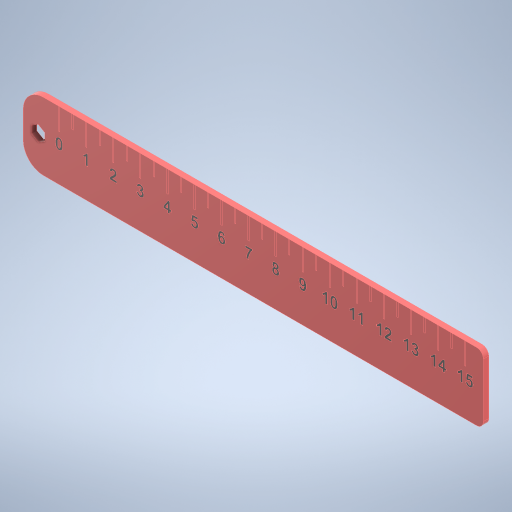
# Autodesk Inventor part: Regua
Saved by Autodesk Inventor 2023 (Build 270158000, 158)
## iProperties
Created: 2024-09-26
Part Number: Regua
Material: Acrílico
Document SubType Name: Modeling
Designer: Aluno
Density: 1.188 g/cm^3
Appearance: Suave - Vermelho
Author: Aluno
Autodesk Inventor part; units mm, degrees
ref_plane "YZ Plane" through (0, 0, 0) normal (1, 0, 0) x (0, 1, 0)
ref_plane "XZ Plane" through (0, 0, 0) normal (0, 1, 0) x (-1, 0, 0)
ref_plane "XY Plane" through (0, 0, 0) normal (0, 0, 1) x (1, 0, 0)
sketch "Esboço1" plane through (0, 0, 0) normal (0, 0, 1) x (1, 0, 0)
  line L0 (-85, 12.5) -> (85, 12.5)
  line L1 (85, 12.5) -> (85, -12.5)
  line L2 (85, -12.5) -> (-85, -12.5)
  line L3 (-85, -12.5) -> (-85, 12.5)
  point P0 (0, 0)
  point P1 (-85, 0)
  point P2 (0, 12.5)
  dimension "d0" = 170
  dimension "d1" = 25
  constraints: 8 end point, 2 midpoint, 2 parallel, 1 horizontal, 1 horizontal alignment, 1 perpendicular, 1 vertical alignment
  measures "d0" distance of L0.start L0.end
  measures "d1" distance of L0.end L1.end
extrude "Extrusão1" add sketch "Esboço1" along normal mid plane 2
fillet "Arredondamento3" radius 7.5 2 edges at (-85, -12.5, 0) (-85, 12.5, 0)
sketch "Esboço3" plane through (0, 0, 1) normal (0, 0, 1) x (1, 0, 0)
  line L0 (-72, 12.5) -> (-71.5, 12.5)
  line L1 (-71.5, 12.5) -> (-71.5, 4.5)
  line L2 (-71.5, 4.5) -> (-72, 4.5)
  line L3 (-72, 4.5) -> (-72, 12.5)
  line L4 (85, 12.5) -> (-77.5, 12.5) projected
  line L5 (-85, 5) -> (-85, -5) projected
  line L6 (-77.5, 12.5) -> (85, 12.5) projected
  line L7 (-67, 12.5) -> (-66.5, 12.5)
  line L8 (-66.5, 12.5) -> (-66.5, 7.5)
  line L9 (-66.5, 7.5) -> (-67, 7.5)
  line L10 (-67, 7.5) -> (-67, 12.5)
  point P0 (0, 0)
  point P1 (72.75, 12.5)
  point P2 (-71.75, 12.5)
  point P3 (-2.375, 12.5)
  point P4 (-66.75, 12.5)
  dimension "d11" = 0.5
  dimension "d12" = 8
  dimension "d13" = 13
  dimension "d14" = 5
  dimension "d15" = 5
  constraints: 16 end point, 5 parallel, 2 horizontal, 2 midpoint, 2 perpendicular, 2 point on line, 1 horizontal alignment
  measures "d11" distance between parallel lines of L3 L1
  measures "d12" distance of L2.end L0.start
  measures "d13" distance between parallel lines of L5 L3
  measures "d14" distance of L9.end L7.start
  measures "d15" distance of point (-71.75, 12.5) point (-66.75, 12.5)
extrude "Extrusão3" cut sketch "Esboço3" against normal blind 0.001
pattern_linear "Padrão retangular1" count 16 spacing 10 along (1, 0, 0) of "Extrusão3"
sketch "Esboço5" plane through (0, 0, 1) normal (0, 0, 1) x (1, 0, 0)
  line L0 (-77, -1.4434) -> (-79.5, -2.8868)
  line L1 (-79.5, -2.8868) -> (-82, -1.4434)
  line L2 (-82, -1.4434) -> (-82, 1.4434)
  line L3 (-82, 1.4434) -> (-79.5, 2.8868)
  line L4 (-79.5, 2.8868) -> (-77, 1.4434)
  line L5 (-77, 1.4434) -> (-77, -1.4434)
  line L6 (-85, 5) -> (-85, -5) projected
  point P0 (0, 0)
  point P1 (-79.5, 0)
  dimension "d23" = 5
  dimension "d24" = 5.5
  constraints: 12 end point, 1 horizontal alignment, 1 vertical alignment, 13 other
  measures "d23" distance between parallel lines of L2 L5
  measures "d24" distance from line of L6 point (-79.5, 0)
extrude "Extrusão5" cut sketch "Esboço5" against normal up to surface (2 mm away)
sketch "Esboço7" plane through (0, 0, 1) normal (0, 0, 1) x (1, 0, 0)
  line L0 (-74.25, 2.5) -> (-69.25, 2.5) construction
  line L1 (-69.25, 2.5) -> (-69.25, -1.5) construction
  line L2 (-69.25, -1.5) -> (-74.25, -1.5) construction
  line L3 (-74.25, -1.5) -> (-74.25, 2.5) construction
  line L4 (-71.5, 4.5) -> (-72, 4.5) projected
  line L5 (-64.25, 2.5) -> (-59.25, 2.5) construction
  line L6 (-59.25, 2.5) -> (-59.25, -1.5) construction
  line L7 (-59.25, -1.5) -> (-64.25, -1.5) construction
  line L8 (-64.25, -1.5) -> (-64.25, 2.5) construction
  line L9 (-54.25, 2.5) -> (-49.25, 2.5) construction
  line L10 (-49.25, 2.5) -> (-49.25, -1.5) construction
  line L11 (-49.25, -1.5) -> (-54.25, -1.5) construction
  line L12 (-54.25, -1.5) -> (-54.25, 2.5) construction
  line L13 (-44.25, 2.5) -> (-39.25, 2.5) construction
  line L14 (-39.25, 2.5) -> (-39.25, -1.5) construction
  line L15 (-39.25, -1.5) -> (-44.25, -1.5) construction
  line L16 (-44.25, -1.5) -> (-44.25, 2.5) construction
  line L17 (-34.25, -1.5) -> (-34.25, 2.5) construction
  line L18 (-34.25, 2.5) -> (-29.25, 2.5) construction
  line L19 (-29.25, 2.5) -> (-29.25, -1.5) construction
  line L20 (-29.25, -1.5) -> (-34.25, -1.5) construction
  line L21 (-24.25, -1.5) -> (-24.25, 2.5) construction
  line L22 (-24.25, 2.5) -> (-19.25, 2.5) construction
  line L23 (-19.25, 2.5) -> (-19.25, -1.5) construction
  line L24 (-19.25, -1.5) -> (-24.25, -1.5) construction
  line L25 (-14.25, -1.5) -> (-14.25, 2.5) construction
  line L26 (-14.25, 2.5) -> (-9.25, 2.5) construction
  line L27 (-9.25, 2.5) -> (-9.25, -1.5) construction
  line L28 (-9.25, -1.5) -> (-14.25, -1.5) construction
  line L29 (-4.25, -1.5) -> (-4.25, 2.5) construction
  line L30 (-4.25, 2.5) -> (0.75, 2.5) construction
  line L31 (0.75, 2.5) -> (0.75, -1.5) construction
  line L32 (0.75, -1.5) -> (-4.25, -1.5) construction
  line L33 (5.75, -1.5) -> (5.75, 2.5) construction
  line L34 (5.75, 2.5) -> (10.75, 2.5) construction
  line L35 (10.75, 2.5) -> (10.75, -1.5) construction
  line L36 (10.75, -1.5) -> (5.75, -1.5) construction
  line L37 (15.75, -1.5) -> (15.75, 2.5) construction
  line L38 (15.75, 2.5) -> (20.75, 2.5) construction
  line L39 (20.75, 2.5) -> (20.75, -1.5) construction
  line L40 (20.75, -1.5) -> (15.75, -1.5) construction
  line L41 (25.75, -1.5) -> (25.75, 2.5) construction
  line L42 (25.75, 2.5) -> (30.75, 2.5) construction
  line L43 (30.75, 2.5) -> (30.75, -1.5) construction
  line L44 (30.75, -1.5) -> (25.75, -1.5) construction
  line L45 (35.75, -1.5) -> (35.75, 2.5) construction
  line L46 (35.75, 2.5) -> (40.75, 2.5) construction
  line L47 (40.75, 2.5) -> (40.75, -1.5) construction
  line L48 (40.75, -1.5) -> (35.75, -1.5) construction
  line L49 (45.75, -1.5) -> (45.75, 2.5) construction
  line L50 (45.75, 2.5) -> (50.75, 2.5) construction
  line L51 (50.75, 2.5) -> (50.75, -1.5) construction
  line L52 (50.75, -1.5) -> (45.75, -1.5) construction
  line L53 (55.75, -1.5) -> (55.75, 2.5) construction
  line L54 (55.75, 2.5) -> (60.75, 2.5) construction
  line L55 (60.75, 2.5) -> (60.75, -1.5) construction
  line L56 (60.75, -1.5) -> (55.75, -1.5) construction
  line L57 (65.75, -1.5) -> (65.75, 2.5) construction
  line L58 (65.75, 2.5) -> (70.75, 2.5) construction
  line L59 (70.75, 2.5) -> (70.75, -1.5) construction
  line L60 (70.75, -1.5) -> (65.75, -1.5) construction
  line L61 (68.5, 4.5) -> (68, 4.5) projected
  line L62 (58.5, 4.5) -> (58, 4.5) projected
  line L63 (48.5, 4.5) -> (48, 4.5) projected
  line L64 (38.5, 4.5) -> (38, 4.5) projected
  line L65 (28.5, 4.5) -> (28, 4.5) projected
  line L66 (18.5, 4.5) -> (18, 4.5) projected
  line L67 (8.5, 4.5) -> (8, 4.5) projected
  line L68 (-1.5, 4.5) -> (-2, 4.5) projected
  line L69 (-11.5, 4.5) -> (-12, 4.5) projected
  line L70 (-21.5, 4.5) -> (-22, 4.5) projected
  line L71 (75.75, -1.5) -> (75.75, 2.5) construction
  line L72 (75.75, 2.5) -> (80.75, 2.5) construction
  line L73 (80.75, 2.5) -> (80.75, -1.5) construction
  line L74 (80.75, -1.5) -> (75.75, -1.5) construction
  line L75 (78.5, 4.5) -> (78, 4.5) projected
  line L76 (-61.5, 4.5) -> (-62, 4.5) projected
  line L77 (-51.5, 4.5) -> (-52, 4.5) projected
  line L78 (-41.5, 4.5) -> (-42, 4.5) projected
  line L79 (-31.5, 4.5) -> (-32, 4.5) projected
  spline S0 degree 2 poles (-71.7698, 2.5412) (-71.1875, 2.5412) (-70.8613, 2.1265) knots 0 0 0 1 1 1
  spline S1 degree 2 poles (-70.8613, 2.1265) (-70.471, 1.6357) (-70.471, 0.4985) knots 0 0 0 1 1 1
  spline S2 degree 2 poles (-70.471, 0.4985) (-70.471, -0.6357) (-70.8643, -1.1326) knots 0 0 0 1 1 1
  spline S3 degree 2 poles (-70.8643, -1.1326) (-71.1875, -1.5412) (-71.7698, -1.5412) knots 0 0 0 1 1 1
  spline S4 degree 2 poles (-71.7698, -1.5412) (-72.3552, -1.5412) (-73.0686, -0.6448) (-73.0686, 0.5076) knots 0 0 0 1 2 2 2
  spline S5 degree 2 poles (-73.0686, 0.5076) (-73.0686, 1.6357) (-72.6753, 2.1326) knots 0 0 0 1 1 1
  spline S6 degree 2 poles (-72.6753, 2.1326) (-72.3521, 2.5412) (-71.7698, 2.5412) knots 0 0 0 1 1 1
  spline S7 degree 2 poles (-71.7698, 1.904) (-71.9101, 1.904) (-72.1265, 1.7271) (-72.1875, 1.4985) knots 0 0 0 1 2 2 2
  spline S8 degree 2 poles (-72.1875, 1.4985) (-72.2668, 1.2027) (-72.2668, 0.4985) knots 0 0 0 1 1 1
  spline S9 degree 2 poles (-72.2668, 0.4985) (-72.2668, -0.2027) (-72.1235, -0.7302) (-71.9101, -0.904) (-71.7698, -0.904) knots 0 0 0 1 2 3 3 3
  spline S10 degree 2 poles (-71.7698, -0.904) (-71.6296, -0.904) (-71.4131, -0.7271) (-71.3521, -0.4985) knots 0 0 0 1 2 2 2
  spline S11 degree 2 poles (-71.3521, -0.4985) (-71.2729, -0.2027) (-71.2729, 0.4985) knots 0 0 0 1 1 1
  spline S12 degree 2 poles (-71.2729, 0.4985) (-71.2729, 1.2027) (-71.4162, 1.7271) (-71.6296, 1.904) (-71.7698, 1.904) knots 0 0 0 1 2 3 3 3
  line L80 (-61.1021, -1.5076) -> (-61.8704, -1.5076)
  line L81 (-61.8704, -1.5076) -> (-61.8704, 1.3796)
  spline S13 degree 2 poles (-61.8704, 1.3796) (-62.2912, 0.9893) (-62.8613, 0.8003) knots 0 0 0 1 1 1
  line L82 (-62.8613, 0.8003) -> (-62.8613, 1.4954)
  spline S14 degree 2 poles (-62.8613, 1.4954) (-62.5595, 1.593) (-61.8552, 2.1418) (-61.7241, 2.5076) knots 0 0 0 1 2 2 2
  line L83 (-61.7241, 2.5076) -> (-61.1021, 2.5076)
  line L84 (-61.1021, 2.5076) -> (-61.1021, -1.5076)
  line L85 (-50.4771, -0.7942) -> (-50.4771, -1.5076)
  line L86 (-50.4771, -1.5076) -> (-53.1631, -1.5076)
  spline S15 degree 2 poles (-53.1631, -1.5076) (-53.1204, -1.1052) (-52.6845, -0.3826) (-52.0381, 0.2149) knots 0 0 0 1 2 2 2
  spline S16 degree 2 poles (-52.0381, 0.2149) (-51.5198, 0.6966) (-51.404, 0.8704) knots 0 0 0 1 1 1
  spline S17 degree 2 poles (-51.404, 0.8704) (-51.2454, 1.1082) (-51.2454, 1.3399) knots 0 0 0 1 1 1
  spline S18 degree 2 poles (-51.2454, 1.3399) (-51.2454, 1.596) (-51.5198, 1.8704) (-51.7637, 1.8704) knots 0 0 0 1 2 2 2
  spline S19 degree 2 poles (-51.7637, 1.8704) (-52.0015, 1.8704) (-52.2851, 1.5808) (-52.3064, 1.2454) knots 0 0 0 1 2 2 2
  line L87 (-52.3064, 1.2454) -> (-53.0716, 1.3216)
  spline S20 degree 2 poles (-53.0716, 1.3216) (-53.0046, 1.9558) (-52.2851, 2.5076) (-51.7454, 2.5076) knots 0 0 0 1 2 2 2
  spline S21 degree 2 poles (-51.7454, 2.5076) (-51.154, 2.5076) (-50.4771, 1.8704) (-50.4771, 1.3948) knots 0 0 0 1 2 2 2
  spline S22 degree 2 poles (-50.4771, 1.3948) (-50.4771, 1.1265) (-50.6692, 0.6387) (-50.8796, 0.3704) knots 0 0 0 1 2 2 2
  spline S23 degree 2 poles (-50.8796, 0.3704) (-51.0198, 0.1936) (-51.7454, -0.471) (-51.9405, -0.6905) (-51.9985, -0.7942) knots 0 0 0 1 2 3 3 3
  line L88 (-51.9985, -0.7942) -> (-50.4771, -0.7942)
  line L89 (-43.093, -0.4101) -> (-42.3521, -0.3186)
  spline S24 degree 2 poles (-42.3521, -0.3186) (-42.3155, -0.6021) (-42.0046, -0.904) (-41.7851, -0.904) knots 0 0 0 1 2 2 2
  spline S25 degree 2 poles (-41.7851, -0.904) (-41.5473, -0.904) (-41.2241, -0.5442) (-41.2241, -0.2393) knots 0 0 0 1 2 2 2
  spline S26 degree 2 poles (-41.2241, -0.2393) (-41.2241, 0.0503) (-41.532, 0.3887) (-41.7546, 0.3887) knots 0 0 0 1 2 2 2
  spline S27 degree 2 poles (-41.7546, 0.3887) (-41.9009, 0.3887) (-42.1052, 0.3308) knots 0 0 0 1 1 1
  line L90 (-42.1052, 0.3308) -> (-42.0198, 0.9558)
  spline S28 degree 2 poles (-42.0198, 0.9558) (-41.7088, 0.9466) (-41.3826, 1.2332) (-41.3826, 1.471) knots 0 0 0 1 2 2 2
  spline S29 degree 2 poles (-41.3826, 1.471) (-41.3826, 1.6723) (-41.6235, 1.9101) (-41.8216, 1.9101) knots 0 0 0 1 2 2 2
  spline S30 degree 2 poles (-41.8216, 1.9101) (-42.0198, 1.9101) (-42.2973, 1.6387) (-42.3277, 1.3765) knots 0 0 0 1 2 2 2
  line L91 (-42.3277, 1.3765) -> (-43.0351, 1.4954)
  spline S31 degree 2 poles (-43.0351, 1.4954) (-42.9619, 1.8582) (-42.6631, 2.2942) (-42.1326, 2.5412) (-41.8003, 2.5412) knots 0 0 0 1 2 3 3 3
  spline S32 degree 2 poles (-41.8003, 2.5412) (-41.2363, 2.5412) (-40.8948, 2.1814) knots 0 0 0 1 1 1
  spline S33 degree 2 poles (-40.8948, 2.1814) (-40.6143, 1.8887) (-40.6143, 1.5168) knots 0 0 0 1 1 1
  spline S34 degree 2 poles (-40.6143, 1.5168) (-40.6143, 0.9924) (-41.1905, 0.6784) knots 0 0 0 1 1 1
  spline S35 degree 2 poles (-41.1905, 0.6784) (-40.846, 0.6052) (-40.4375, 0.0899) (-40.4375, -0.2729) knots 0 0 0 1 2 2 2
  spline S36 degree 2 poles (-40.4375, -0.2729) (-40.4375, -0.8003) (-41.2058, -1.5412) (-41.779, -1.5412) knots 0 0 0 1 2 2 2
  spline S37 degree 2 poles (-41.779, -1.5412) (-42.3216, -1.5412) (-43.0351, -0.9162) (-43.093, -0.4101) knots 0 0 0 1 2 2 2
  line L92 (-31.5625, -1.5076) -> (-31.5625, -0.7027)
  line L93 (-31.5625, -0.7027) -> (-33.1997, -0.7027)
  line L94 (-33.1997, -0.7027) -> (-33.1997, -0.0351)
  line L95 (-33.1997, -0.0351) -> (-31.4649, 2.5076)
  line L96 (-31.4649, 2.5076) -> (-30.8216, 2.5076)
  line L97 (-30.8216, 2.5076) -> (-30.8216, -0.032)
  line L98 (-30.8216, -0.032) -> (-30.3247, -0.032)
  line L99 (-30.3247, -0.032) -> (-30.3247, -0.7027)
  line L100 (-30.3247, -0.7027) -> (-30.8216, -0.7027)
  line L101 (-30.8216, -0.7027) -> (-30.8216, -1.5076)
  line L102 (-30.8216, -1.5076) -> (-31.5625, -1.5076)
  line L103 (-31.5625, -0.032) -> (-31.5625, 1.3369)
  line L104 (-31.5625, 1.3369) -> (-32.4832, -0.032)
  line L105 (-32.4832, -0.032) -> (-31.5625, -0.032)
  line L106 (-23.0564, -0.4131) -> (-22.2912, -0.3338)
  spline S38 degree 2 poles (-22.2912, -0.3338) (-22.2576, -0.593) (-21.9375, -0.8948) (-21.7271, -0.8948) knots 0 0 0 1 2 2 2
  spline S39 degree 2 poles (-21.7271, -0.8948) (-21.4863, -0.8948) (-21.154, -0.5046) (-21.154, -0.1082) knots 0 0 0 1 2 2 2
  spline S40 degree 2 poles (-21.154, -0.1082) (-21.154, 0.2607) (-21.4863, 0.6296) (-21.7515, 0.6296) knots 0 0 0 1 2 2 2
  spline S41 degree 2 poles (-21.7515, 0.6296) (-22.0808, 0.6296) (-22.343, 0.3369) knots 0 0 0 1 1 1
  line L107 (-22.343, 0.3369) -> (-22.9649, 0.4284)
  line L108 (-22.9649, 0.4284) -> (-22.5716, 2.5076)
  line L109 (-22.5716, 2.5076) -> (-20.5412, 2.5076)
  line L110 (-20.5412, 2.5076) -> (-20.5412, 1.7912)
  line L111 (-20.5412, 1.7912) -> (-21.9893, 1.7912)
  line L112 (-21.9893, 1.7912) -> (-22.1113, 1.1113)
  spline S42 degree 2 poles (-22.1113, 1.1113) (-21.8552, 1.2393) (-21.5869, 1.2393) knots 0 0 0 1 1 1
  spline S43 degree 2 poles (-21.5869, 1.2393) (-21.0747, 1.2393) (-20.3643, 0.4954) (-20.3643, -0.096) knots 0 0 0 1 2 2 2
  spline S44 degree 2 poles (-20.3643, -0.096) (-20.3643, -0.5899) (-20.6509, -0.9771) knots 0 0 0 1 1 1
  spline S45 degree 2 poles (-20.6509, -0.9771) (-21.0412, -1.5076) (-21.7363, -1.5076) knots 0 0 0 1 1 1
  spline S46 degree 2 poles (-21.7363, -1.5076) (-22.2881, -1.5076) (-22.9893, -0.9131) (-23.0564, -0.4131) knots 0 0 0 1 2 2 2
  line L113 (-10.468, 1.5473) -> (-11.2088, 1.4649)
  spline S47 degree 2 poles (-11.2088, 1.4649) (-11.2363, 1.6936) (-11.4649, 1.9101) (-11.6479, 1.9101) knots 0 0 0 1 2 2 2
  spline S48 degree 2 poles (-11.6479, 1.9101) (-11.8918, 1.9101) (-12.2271, 1.4741) (-12.2698, 0.7851) knots 0 0 0 1 2 2 2
  spline S49 degree 2 poles (-12.2698, 0.7851) (-11.9863, 1.1235) (-11.5595, 1.1235) knots 0 0 0 1 1 1
  spline S50 degree 2 poles (-11.5595, 1.1235) (-11.0808, 1.1235) (-10.3948, 0.3918) (-10.3948, -0.1845) knots 0 0 0 1 2 2 2
  spline S51 degree 2 poles (-10.3948, -0.1845) (-10.3948, -0.8003) (-11.1143, -1.5412) (-11.6784, -1.5412) knots 0 0 0 1 2 2 2
  spline S52 degree 2 poles (-11.6784, -1.5412) (-12.2851, -1.5412) (-13.0655, -0.5991) (-13.0655, 0.471) knots 0 0 0 1 2 2 2
  spline S53 degree 2 poles (-13.0655, 0.471) (-13.0655, 1.5716) (-12.2515, 2.5412) (-11.6021, 2.5412) knots 0 0 0 1 2 2 2
  spline S54 degree 2 poles (-11.6021, 2.5412) (-11.1479, 2.5412) (-10.5503, 2.032) (-10.468, 1.5473) knots 0 0 0 1 2 2 2
  spline S55 degree 2 poles (-12.2058, -0.1235) (-12.2058, -0.4985) (-11.8613, -0.904) (-11.6418, -0.904) knots 0 0 0 1 2 2 2
  spline S56 degree 2 poles (-11.6418, -0.904) (-11.4284, -0.904) (-11.1448, -0.5716) (-11.1448, -0.1936) knots 0 0 0 1 2 2 2
  spline S57 degree 2 poles (-11.1448, -0.1936) (-11.1448, 0.1966) (-11.4497, 0.5595) (-11.6784, 0.5595) knots 0 0 0 1 2 2 2
  spline S58 degree 2 poles (-11.6784, 0.5595) (-11.9009, 0.5595) (-12.2058, 0.2119) (-12.2058, -0.1235) knots 0 0 0 1 2 2 2
  line L114 (-3.0655, 1.7607) -> (-3.0655, 2.4741)
  line L115 (-3.0655, 2.4741) -> (-0.4436, 2.4741)
  line L116 (-0.4436, 2.4741) -> (-0.4436, 1.9162)
  spline S59 degree 2 poles (-0.4436, 1.9162) (-0.7668, 1.596) (-1.4375, 0.4009) (-1.7912, -0.9436) (-1.7881, -1.4741) knots 0 0 0 1 2 3 3 3
  line L117 (-1.7881, -1.4741) -> (-2.529, -1.4741)
  spline S60 degree 2 poles (-2.529, -1.4741) (-2.5107, -0.6448) (-1.8613, 1.0808) (-1.3216, 1.7607) knots 0 0 0 1 2 2 2
  line L118 (-1.3216, 1.7607) -> (-3.0655, 1.7607)
  spline S61 degree 2 poles (7.5899, 0.686) (7.2942, 0.811) (7.0229, 1.25) (7.0229, 1.5122) knots 0 0 0 1 2 2 2
  spline S62 degree 2 poles (7.0229, 1.5122) (7.0229, 1.9604) (7.6479, 2.5427) (8.2241, 2.5427) knots 0 0 0 1 2 2 2
  spline S63 degree 2 poles (8.2241, 2.5427) (8.7942, 2.5427) (9.4253, 1.9604) (9.4253, 1.5122) knots 0 0 0 1 2 2 2
  spline S64 degree 2 poles (9.4253, 1.5122) (9.4253, 1.2348) (9.1357, 0.8018) (8.8735, 0.686) knots 0 0 0 1 2 2 2
  spline S65 degree 2 poles (8.8735, 0.686) (9.2058, 0.5518) (9.5534, 0.0396) (9.5534, -0.2957) knots 0 0 0 1 2 2 2
  spline S66 degree 2 poles (9.5534, -0.2957) (9.5534, -0.8506) (8.846, -1.5427) (8.2607, -1.5427) knots 0 0 0 1 2 2 2
  spline S67 degree 2 poles (8.2607, -1.5427) (7.7149, -1.5427) (7.3521, -1.2561) knots 0 0 0 1 1 1
  spline S68 degree 2 poles (7.3521, -1.2561) (6.9223, -0.9177) (6.9223, -0.3293) knots 0 0 0 1 1 1
  spline S69 degree 2 poles (6.9223, -0.3293) (6.9223, -0.003) (7.2454, 0.5396) (7.5899, 0.686) knots 0 0 0 1 2 2 2
  spline S70 degree 2 poles (7.6784, -0.2561) (7.6784, -0.5732) (8.0015, -0.9268) (8.2454, -0.9268) knots 0 0 0 1 2 2 2
  spline S71 degree 2 poles (8.2454, -0.9268) (8.4832, -0.9268) (8.7942, -0.5854) (8.7942, -0.2622) knots 0 0 0 1 2 2 2
  spline S72 degree 2 poles (8.7942, -0.2622) (8.7942, 0.0183) (8.4771, 0.3598) (8.2363, 0.3598) knots 0 0 0 1 2 2 2
  spline S73 degree 2 poles (8.2363, 0.3598) (7.9527, 0.3598) (7.6784, -0.0274) (7.6784, -0.2561) knots 0 0 0 1 2 2 2
  spline S74 degree 2 poles (7.7485, 1.4573) (7.7485, 1.2287) (8.0076, 0.9726) (8.2241, 0.9726) knots 0 0 0 1 2 2 2
  spline S75 degree 2 poles (8.2241, 0.9726) (8.4436, 0.9726) (8.7058, 1.2317) (8.7058, 1.4604) knots 0 0 0 1 2 2 2
  spline S76 degree 2 poles (8.7058, 1.4604) (8.7058, 1.6738) (8.4466, 1.9329) (8.2332, 1.9329) knots 0 0 0 1 2 2 2
  spline S77 degree 2 poles (8.2332, 1.9329) (8.0107, 1.9329) (7.7485, 1.6707) (7.7485, 1.4573) knots 0 0 0 1 2 2 2
  line L119 (16.9497, -0.5427) -> (17.6905, -0.4604)
  spline S78 degree 2 poles (17.6905, -0.4604) (17.718, -0.686) (17.9466, -0.9055) (18.1357, -0.9055) knots 0 0 0 1 2 2 2
  spline S79 degree 2 poles (18.1357, -0.9055) (18.3735, -0.9055) (18.7058, -0.4695) (18.7515, 0.2195) knots 0 0 0 1 2 2 2
  spline S80 degree 2 poles (18.7515, 0.2195) (18.4649, -0.1159) (18.029, -0.1159) knots 0 0 0 1 1 1
  spline S81 degree 2 poles (18.029, -0.1159) (17.5595, -0.1159) (16.8735, 0.6098) (16.8735, 1.1921) knots 0 0 0 1 2 2 2
  spline S82 degree 2 poles (16.8735, 1.1921) (16.8735, 1.7988) (17.596, 2.5427) (18.157, 2.5427) knots 0 0 0 1 2 2 2
  spline S83 degree 2 poles (18.157, 2.5427) (18.7637, 2.5427) (19.5442, 1.6006) (19.5442, 0.5244) knots 0 0 0 1 2 2 2
  spline S84 degree 2 poles (19.5442, 0.5244) (19.5442, -0.5732) (18.7302, -1.5427) (18.0777, -1.5427) knots 0 0 0 1 2 2 2
  spline S85 degree 2 poles (18.0777, -1.5427) (17.6113, -1.5427) (17.032, -1.0396) (16.9497, -0.5427) knots 0 0 0 1 2 2 2
  spline S86 degree 2 poles (18.6845, 1.128) (18.6845, 1.497) (18.343, 1.9055) (18.1204, 1.9055) knots 0 0 0 1 2 2 2
  spline S87 degree 2 poles (18.1204, 1.9055) (17.907, 1.9055) (17.6265, 1.5701) (17.6265, 1.1921) knots 0 0 0 1 2 2 2
  spline S88 degree 2 poles (17.6265, 1.1921) (17.6265, 0.8049) (17.9314, 0.4451) (18.1601, 0.4451) knots 0 0 0 1 2 2 2
  spline S89 degree 2 poles (18.1601, 0.4451) (18.3826, 0.4451) (18.6845, 0.7927) (18.6845, 1.128) knots 0 0 0 1 2 2 2
  line L120 (27.3445, -1.4741) -> (26.5762, -1.4741)
  line L121 (26.5762, -1.4741) -> (26.5762, 1.4131)
  spline S90 degree 2 poles (26.5762, 1.4131) (26.1555, 1.0229) (25.5854, 0.8338) knots 0 0 0 1 1 1
  line L122 (25.5854, 0.8338) -> (25.5854, 1.529)
  spline S91 degree 2 poles (25.5854, 1.529) (25.8872, 1.6265) (26.5915, 2.1753) (26.7226, 2.5412) knots 0 0 0 1 2 2 2
  line L123 (26.7226, 2.5412) -> (27.3445, 2.5412)
  line L124 (27.3445, 2.5412) -> (27.3445, -1.4741)
  spline S92 degree 2 poles (29.7835, 2.5412) (30.3659, 2.5412) (30.6921, 2.1265) knots 0 0 0 1 1 1
  spline S93 degree 2 poles (30.6921, 2.1265) (31.0823, 1.6357) (31.0823, 0.4985) knots 0 0 0 1 1 1
  spline S94 degree 2 poles (31.0823, 0.4985) (31.0823, -0.6357) (30.689, -1.1326) knots 0 0 0 1 1 1
  spline S95 degree 2 poles (30.689, -1.1326) (30.3659, -1.5412) (29.7835, -1.5412) knots 0 0 0 1 1 1
  spline S96 degree 2 poles (29.7835, -1.5412) (29.1982, -1.5412) (28.4848, -0.6448) (28.4848, 0.5076) knots 0 0 0 1 2 2 2
  spline S97 degree 2 poles (28.4848, 0.5076) (28.4848, 1.6357) (28.878, 2.1326) knots 0 0 0 1 1 1
  spline S98 degree 2 poles (28.878, 2.1326) (29.2012, 2.5412) (29.7835, 2.5412) knots 0 0 0 1 1 1
  spline S99 degree 2 poles (29.7835, 1.904) (29.6433, 1.904) (29.4268, 1.7271) (29.3659, 1.4985) knots 0 0 0 1 2 2 2
  spline S100 degree 2 poles (29.3659, 1.4985) (29.2866, 1.2027) (29.2866, 0.4985) knots 0 0 0 1 1 1
  spline S101 degree 2 poles (29.2866, 0.4985) (29.2866, -0.2027) (29.4299, -0.7302) (29.6433, -0.904) (29.7835, -0.904) knots 0 0 0 1 2 3 3 3
  spline S102 degree 2 poles (29.7835, -0.904) (29.9238, -0.904) (30.1402, -0.7271) (30.2012, -0.4985) knots 0 0 0 1 2 2 2
  spline S103 degree 2 poles (30.2012, -0.4985) (30.2805, -0.2027) (30.2805, 0.4985) knots 0 0 0 1 1 1
  spline S104 degree 2 poles (30.2805, 0.4985) (30.2805, 1.2027) (30.1372, 1.7271) (29.9238, 1.904) (29.7835, 1.904) knots 0 0 0 1 2 3 3 3
  line L125 (37.3445, -1.5076) -> (36.5762, -1.5076)
  line L126 (36.5762, -1.5076) -> (36.5762, 1.3796)
  spline S105 degree 2 poles (36.5762, 1.3796) (36.1555, 0.9893) (35.5854, 0.8003) knots 0 0 0 1 1 1
  line L127 (35.5854, 0.8003) -> (35.5854, 1.4954)
  spline S106 degree 2 poles (35.5854, 1.4954) (35.8872, 1.593) (36.5915, 2.1418) (36.7226, 2.5076) knots 0 0 0 1 2 2 2
  line L128 (36.7226, 2.5076) -> (37.3445, 2.5076)
  line L129 (37.3445, 2.5076) -> (37.3445, -1.5076)
  line L130 (40.4512, -1.5076) -> (39.6829, -1.5076)
  line L131 (39.6829, -1.5076) -> (39.6829, 1.3796)
  spline S107 degree 2 poles (39.6829, 1.3796) (39.2622, 0.9893) (38.6921, 0.8003) knots 0 0 0 1 1 1
  line L132 (38.6921, 0.8003) -> (38.6921, 1.4954)
  spline S108 degree 2 poles (38.6921, 1.4954) (38.9939, 1.593) (39.6982, 2.1418) (39.8293, 2.5076) knots 0 0 0 1 2 2 2
  line L133 (39.8293, 2.5076) -> (40.4512, 2.5076)
  line L134 (40.4512, 2.5076) -> (40.4512, -1.5076)
  line L135 (47.3445, -1.5076) -> (46.5762, -1.5076)
  line L136 (46.5762, -1.5076) -> (46.5762, 1.3796)
  spline S109 degree 2 poles (46.5762, 1.3796) (46.1555, 0.9893) (45.5854, 0.8003) knots 0 0 0 1 1 1
  line L137 (45.5854, 0.8003) -> (45.5854, 1.4954)
  spline S110 degree 2 poles (45.5854, 1.4954) (45.8872, 1.593) (46.5915, 2.1418) (46.7226, 2.5076) knots 0 0 0 1 2 2 2
  line L138 (46.7226, 2.5076) -> (47.3445, 2.5076)
  line L139 (47.3445, 2.5076) -> (47.3445, -1.5076)
  line L140 (51.0762, -0.7942) -> (51.0762, -1.5076)
  line L141 (51.0762, -1.5076) -> (48.3902, -1.5076)
  spline S111 degree 2 poles (48.3902, -1.5076) (48.4329, -1.1052) (48.8689, -0.3826) (49.5152, 0.2149) knots 0 0 0 1 2 2 2
  spline S112 degree 2 poles (49.5152, 0.2149) (50.0335, 0.6966) (50.1494, 0.8704) knots 0 0 0 1 1 1
  spline S113 degree 2 poles (50.1494, 0.8704) (50.3079, 1.1082) (50.3079, 1.3399) knots 0 0 0 1 1 1
  spline S114 degree 2 poles (50.3079, 1.3399) (50.3079, 1.596) (50.0335, 1.8704) (49.7896, 1.8704) knots 0 0 0 1 2 2 2
  spline S115 degree 2 poles (49.7896, 1.8704) (49.5518, 1.8704) (49.2683, 1.5808) (49.247, 1.2454) knots 0 0 0 1 2 2 2
  line L142 (49.247, 1.2454) -> (48.4817, 1.3216)
  spline S116 degree 2 poles (48.4817, 1.3216) (48.5488, 1.9558) (49.2683, 2.5076) (49.8079, 2.5076) knots 0 0 0 1 2 2 2
  spline S117 degree 2 poles (49.8079, 2.5076) (50.3994, 2.5076) (51.0762, 1.8704) (51.0762, 1.3948) knots 0 0 0 1 2 2 2
  spline S118 degree 2 poles (51.0762, 1.3948) (51.0762, 1.1265) (50.8841, 0.6387) (50.6738, 0.3704) knots 0 0 0 1 2 2 2
  spline S119 degree 2 poles (50.6738, 0.3704) (50.5335, 0.1936) (49.8079, -0.471) (49.6128, -0.6905) (49.5549, -0.7942) knots 0 0 0 1 2 3 3 3
  line L143 (49.5549, -0.7942) -> (51.0762, -0.7942)
  line L144 (57.3445, -1.4741) -> (56.5762, -1.4741)
  line L145 (56.5762, -1.4741) -> (56.5762, 1.4131)
  spline S120 degree 2 poles (56.5762, 1.4131) (56.1555, 1.0229) (55.5854, 0.8338) knots 0 0 0 1 1 1
  line L146 (55.5854, 0.8338) -> (55.5854, 1.529)
  spline S121 degree 2 poles (55.5854, 1.529) (55.8872, 1.6265) (56.5915, 2.1753) (56.7226, 2.5412) knots 0 0 0 1 2 2 2
  line L147 (56.7226, 2.5412) -> (57.3445, 2.5412)
  line L148 (57.3445, 2.5412) -> (57.3445, -1.4741)
  line L149 (58.4604, -0.4101) -> (59.2012, -0.3186)
  spline S122 degree 2 poles (59.2012, -0.3186) (59.2378, -0.6021) (59.5488, -0.904) (59.7683, -0.904) knots 0 0 0 1 2 2 2
  spline S123 degree 2 poles (59.7683, -0.904) (60.0061, -0.904) (60.3293, -0.5442) (60.3293, -0.2393) knots 0 0 0 1 2 2 2
  spline S124 degree 2 poles (60.3293, -0.2393) (60.3293, 0.0503) (60.0213, 0.3887) (59.7988, 0.3887) knots 0 0 0 1 2 2 2
  spline S125 degree 2 poles (59.7988, 0.3887) (59.6524, 0.3887) (59.4482, 0.3308) knots 0 0 0 1 1 1
  line L150 (59.4482, 0.3308) -> (59.5335, 0.9558)
  spline S126 degree 2 poles (59.5335, 0.9558) (59.8445, 0.9466) (60.1707, 1.2332) (60.1707, 1.471) knots 0 0 0 1 2 2 2
  spline S127 degree 2 poles (60.1707, 1.471) (60.1707, 1.6723) (59.9299, 1.9101) (59.7317, 1.9101) knots 0 0 0 1 2 2 2
  spline S128 degree 2 poles (59.7317, 1.9101) (59.5335, 1.9101) (59.2561, 1.6387) (59.2256, 1.3765) knots 0 0 0 1 2 2 2
  line L151 (59.2256, 1.3765) -> (58.5183, 1.4954)
  spline S129 degree 2 poles (58.5183, 1.4954) (58.5915, 1.8582) (58.8902, 2.2942) (59.4207, 2.5412) (59.753, 2.5412) knots 0 0 0 1 2 3 3 3
  spline S130 degree 2 poles (59.753, 2.5412) (60.3171, 2.5412) (60.6585, 2.1814) knots 0 0 0 1 1 1
  spline S131 degree 2 poles (60.6585, 2.1814) (60.939, 1.8887) (60.939, 1.5168) knots 0 0 0 1 1 1
  spline S132 degree 2 poles (60.939, 1.5168) (60.939, 0.9924) (60.3628, 0.6784) knots 0 0 0 1 1 1
  spline S133 degree 2 poles (60.3628, 0.6784) (60.7073, 0.6052) (61.1159, 0.0899) (61.1159, -0.2729) knots 0 0 0 1 2 2 2
  spline S134 degree 2 poles (61.1159, -0.2729) (61.1159, -0.8003) (60.3476, -1.5412) (59.7744, -1.5412) knots 0 0 0 1 2 2 2
  spline S135 degree 2 poles (59.7744, -1.5412) (59.2317, -1.5412) (58.5183, -0.9162) (58.4604, -0.4101) knots 0 0 0 1 2 2 2
  line L152 (67.3445, -1.5076) -> (66.5762, -1.5076)
  line L153 (66.5762, -1.5076) -> (66.5762, 1.3796)
  spline S136 degree 2 poles (66.5762, 1.3796) (66.1555, 0.9893) (65.5854, 0.8003) knots 0 0 0 1 1 1
  line L154 (65.5854, 0.8003) -> (65.5854, 1.4954)
  spline S137 degree 2 poles (65.5854, 1.4954) (65.8872, 1.593) (66.5915, 2.1418) (66.7226, 2.5076) knots 0 0 0 1 2 2 2
  line L155 (66.7226, 2.5076) -> (67.3445, 2.5076)
  line L156 (67.3445, 2.5076) -> (67.3445, -1.5076)
  line L157 (69.9909, -1.5076) -> (69.9909, -0.7027)
  line L158 (69.9909, -0.7027) -> (68.3537, -0.7027)
  line L159 (68.3537, -0.7027) -> (68.3537, -0.0351)
  line L160 (68.3537, -0.0351) -> (70.0884, 2.5076)
  line L161 (70.0884, 2.5076) -> (70.7317, 2.5076)
  line L162 (70.7317, 2.5076) -> (70.7317, -0.032)
  line L163 (70.7317, -0.032) -> (71.2287, -0.032)
  line L164 (71.2287, -0.032) -> (71.2287, -0.7027)
  line L165 (71.2287, -0.7027) -> (70.7317, -0.7027)
  line L166 (70.7317, -0.7027) -> (70.7317, -1.5076)
  line L167 (70.7317, -1.5076) -> (69.9909, -1.5076)
  line L168 (69.9909, -0.032) -> (69.9909, 1.3369)
  line L169 (69.9909, 1.3369) -> (69.0701, -0.032)
  line L170 (69.0701, -0.032) -> (69.9909, -0.032)
  line L171 (77.3445, -1.4741) -> (76.5762, -1.4741)
  line L172 (76.5762, -1.4741) -> (76.5762, 1.4131)
  spline S138 degree 2 poles (76.5762, 1.4131) (76.1555, 1.0229) (75.5854, 0.8338) knots 0 0 0 1 1 1
  line L173 (75.5854, 0.8338) -> (75.5854, 1.529)
  spline S139 degree 2 poles (75.5854, 1.529) (75.8872, 1.6265) (76.5915, 2.1753) (76.7226, 2.5412) knots 0 0 0 1 2 2 2
  line L174 (76.7226, 2.5412) -> (77.3445, 2.5412)
  line L175 (77.3445, 2.5412) -> (77.3445, -1.4741)
  line L176 (78.497, -0.4466) -> (79.2622, -0.3674)
  spline S140 degree 2 poles (79.2622, -0.3674) (79.2957, -0.6265) (79.6159, -0.9284) (79.8262, -0.9284) knots 0 0 0 1 2 2 2
  spline S141 degree 2 poles (79.8262, -0.9284) (80.0671, -0.9284) (80.3994, -0.5381) (80.3994, -0.1418) knots 0 0 0 1 2 2 2
  spline S142 degree 2 poles (80.3994, -0.1418) (80.3994, 0.2271) (80.0671, 0.596) (79.8018, 0.596) knots 0 0 0 1 2 2 2
  spline S143 degree 2 poles (79.8018, 0.596) (79.4726, 0.596) (79.2104, 0.3034) knots 0 0 0 1 1 1
  line L177 (79.2104, 0.3034) -> (78.5884, 0.3948)
  line L178 (78.5884, 0.3948) -> (78.9817, 2.4741)
  line L179 (78.9817, 2.4741) -> (81.0122, 2.4741)
  line L180 (81.0122, 2.4741) -> (81.0122, 1.7576)
  line L181 (81.0122, 1.7576) -> (79.564, 1.7576)
  line L182 (79.564, 1.7576) -> (79.4421, 1.0777)
  spline S144 degree 2 poles (79.4421, 1.0777) (79.6982, 1.2058) (79.9665, 1.2058) knots 0 0 0 1 1 1
  spline S145 degree 2 poles (79.9665, 1.2058) (80.4787, 1.2058) (81.189, 0.4619) (81.189, -0.1296) knots 0 0 0 1 2 2 2
  spline S146 degree 2 poles (81.189, -0.1296) (81.189, -0.6235) (80.9024, -1.0107) knots 0 0 0 1 1 1
  spline S147 degree 2 poles (80.9024, -1.0107) (80.5122, -1.5412) (79.8171, -1.5412) knots 0 0 0 1 1 1
  spline S148 degree 2 poles (79.8171, -1.5412) (79.2652, -1.5412) (78.564, -0.9466) (78.497, -0.4466) knots 0 0 0 1 2 2 2
  point P0 (0, 0)
  point P1 (-71.75, 2.5)
  point P2 (-71.75, 4.5)
  point P3 (-61.75, 2.5)
  point P4 (-51.75, 2.5)
  point P5 (-41.75, 2.5)
  point P6 (-31.75, 2.5)
  point P7 (-21.75, 2.5)
  point P8 (-11.75, 2.5)
  point P9 (-1.75, 2.5)
  point P10 (8.25, 2.5)
  point P11 (18.25, 2.5)
  point P12 (28.25, 2.5)
  point P13 (38.25, 2.5)
  point P14 (48.25, 2.5)
  point P15 (58.25, 2.5)
  point P16 (68.25, 2.5)
  point P17 (68.25, 4.5)
  point P18 (58.25, 4.5)
  point P19 (48.25, 4.5)
  point P20 (38.25, 4.5)
  point P21 (28.25, 4.5)
  point P22 (18.25, 4.5)
  point P23 (8.25, 4.5)
  point P24 (-1.75, 4.5)
  point P25 (-11.75, 4.5)
  point P26 (-21.75, 4.5)
  point P27 (78.25, 2.5)
  point P28 (78.25, 4.5)
  point P29 (-61.75, 4.5)
  point P30 (-51.75, 4.5)
  point P31 (-41.75, 4.5)
  point P32 (-31.75, 4.5)
  dimension "d30" = 4
  dimension "d31" = 2
  dimension "d32" = 4
  dimension "d33" = 4
  dimension "d34" = 4
  dimension "d35" = 4
  dimension "d36" = 4
  dimension "d37" = 4
  dimension "d38" = 4
  dimension "d39" = 4
  dimension "d40" = 4
  dimension "d41" = 4
  dimension "d42" = 4
  dimension "d43" = 4
  dimension "d44" = 4
  dimension "d45" = 4
  dimension "d49" = 4
  dimension "d50" = 5
  constraints: 32 midpoint, 30 horizontal alignment, 16 vertical alignment, 15 collinear, 32 other
  measures "d30" distance between parallel lines of L2 L0
  measures "d31" distance between parallel lines of L0 L4
  measures "d32" distance between parallel lines of L7 L5
  measures "d33" distance between parallel lines of L11 L9
  measures "d34" distance between parallel lines of L15 L13
  measures "d35" distance between parallel lines of L20 L18
  measures "d36" distance between parallel lines of L24 L22
  measures "d37" distance between parallel lines of L28 L26
  measures "d38" distance between parallel lines of L32 L30
  measures "d39" distance between parallel lines of L36 L34
  measures "d40" distance between parallel lines of L40 L38
  measures "d41" distance between parallel lines of L44 L42
  measures "d42" distance between parallel lines of L48 L46
  measures "d43" distance between parallel lines of L52 L50
  measures "d44" distance between parallel lines of L56 L54
  measures "d45" distance between parallel lines of L60 L58
  measures "d49" distance between parallel lines of L74 L72
  measures "d50" distance of L1.end L2.end
sketch "Esboço8" plane through (83, 12.5, 0.999) normal (0, 0, 1) x (1, 0, 0)
  line L0 (0.5, 0) -> (0.5, -5) projected
  line L1 (0, 0) -> (0.5, 0) projected
  line L2 (0, -5) -> (0, 0) projected
  line L3 (0.5, -5) -> (0, -5) projected
  point P0 (-83, -12.5)
extrude "Extrusão7" add sketch "Esboço8" along normal up to surface (0.001 mm away)
fillet "Arredondamento5" radius 2.5 2 edges at (85, 12.5, 0) (85, -12.5, 0)
emboss "Relevo1" sketch "Esboço7" operation cut depth 0.01 direction (0, 0, -1)
